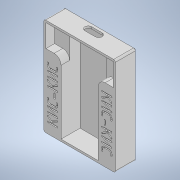
# Autodesk Inventor part: Корпус
Saved by Autodesk Inventor 2021.2 (Build 252289000, 289)
## iProperties
Created: 2023-10-18
Part Number: Корпус
Material: Типовые
Document SubType Name: Modeling
Designer: DELL
Density: 1 g/cm^3
Appearance: По умолчанию
Author: DELL
Autodesk Inventor part; units mm, degrees
ref_plane "YZ Plane" through (0, 0, 0) normal (1, 0, 0) x (0, 1, 0)
ref_plane "XZ Plane" through (0, 0, 0) normal (0, 1, 0) x (-1, 0, 0)
ref_plane "XY Plane" through (0, 0, 0) normal (0, 0, 1) x (1, 0, 0)
sketch "Эскиз1" plane through (0, 0, 0) normal (0, 0, 1) x (1, 0, 0)
  line L0 (10.25, -26.5) -> (-10.25, -26.5) construction
  line L1 (-10.25, -26.5) -> (-10.25, 26.5) construction
  line L2 (-10.25, 26.5) -> (10.25, 26.5) construction
  line L3 (10.25, 26.5) -> (10.25, -26.5) construction
  line L4 (10.25, -26.5) -> (-10.25, 26.5) construction
  line L5 (-10.25, -26.5) -> (10.25, 26.5) construction
  line L6 (19, 14.5) -> (-19, 14.5) construction
  line L7 (-19, 14.5) -> (-19, 26.5) construction
  line L8 (-19, 26.5) -> (19, 26.5) construction
  line L9 (19, 26.5) -> (19, 14.5) construction
  line L10 (19, 14.5) -> (-19, 26.5) construction
  line L11 (-19, 14.5) -> (19, 26.5) construction
  line L12 (-19.5, 14) -> (-14.75, 14)
  arc A0 (-10.75, 10) -> (-14.75, 14) centre (-14.75, 10) ccw
  line L13 (-10.75, 10) -> (-10.75, -27)
  line L14 (-10.75, -27) -> (10.75, -27)
  line L15 (10.75, -27) -> (10.75, 10)
  arc A1 (14.75, 14) -> (10.75, 10) centre (14.75, 10) ccw
  line L16 (14.75, 14) -> (19.5, 14)
  line L17 (19.5, 14) -> (19.5, 27)
  line L18 (19.5, 27) -> (-19.5, 27)
  line L19 (-19.5, 27) -> (-19.5, 14)
  line L20 (0, 26.5) -> (0, -26.5) construction
  line L21 (20.7, -28.2) -> (-20.7, -28.2)
  line L22 (-20.7, -28.2) -> (-20.7, 28.2)
  line L23 (-20.7, 28.2) -> (20.7, 28.2)
  line L24 (20.7, 28.2) -> (20.7, -28.2)
  line L25 (20.7, -28.2) -> (-20.7, 28.2) construction
  line L26 (-20.7, -28.2) -> (20.7, 28.2) construction
  line L27 (-10.75, 10) -> (-10.75, 27)
  line L28 (10.75, 10) -> (10.75, 27)
  point P0 (0, 0)
  point P1 (0, 20.5)
  point P2 (0, 20.5)
  point P3 (0, 0)
  point P4 (0, 0)
  dimension "d0" = 20.5
  dimension "d1" = 53
  dimension "d2" = 38
  dimension "d3" = 12
  dimension "d4" = 0
  dimension "d5" = 0.5
  dimension "d8" = 0.5
  dimension "d9" = 0.5
  dimension "d10" = 0.5
  dimension "d11" = 0.5
  dimension "d12" = 4
  dimension "d13" = 1.2
  dimension "d14" = 1.2
  dimension "d15" = 1.2
  constraints: 58 end point, 11 midpoint, 10 perpendicular, 7 parallel, 5 horizontal, 4 point on circle, 4 tangent, 3 point on line, 2 centre point, 1 vertical alignment, 3 other
  measures "d0" distance of L1.end L2.end
  measures "d1" distance of L0.end L1.end
  measures "d2" distance of L7.end L8.end
  measures "d3" distance of L6.end L7.end
  measures "d4" distance between parallel lines of L2 L8
  measures "d5" distance between parallel lines of L19 L7
  measures "d8" distance between parallel lines of L18 L8
  measures "d9" distance between parallel lines of L6 L12
  measures "d10" distance between parallel lines of L1 L13
  measures "d11" distance between parallel lines of L0 L14
  measures "d12" radius of A0
  measures "d13" distance between parallel lines of L23 L18
  measures "d14" distance between parallel lines of L22 L19
  measures "d15" distance between parallel lines of L14 L21
extrude "Выдавливание1" add sketch "Эскиз1" along normal blind 6 contours L19 L18 L27 A0 L12 | L18 L17 L16 A1 L28 | L21 L22 L23 L24
extrude "Выдавливание2" add sketch "Эскиз1" along normal blind 5 from surface at 6
extrude "Выдавливание3" add sketch "Эскиз1" against normal blind 1 contours L19 L18 L27 A0 L12 | L27 L18 L28 L15 L14 L13 | L18 L17 L16 A1 L28 | L21 L22 L23 L24
fillet "Сопряжение1" radius 1 4 edges at (-20.7, 28.2, 5) (20.7, 28.2, 5) (-20.7, -28.2, 5) (20.7, -28.2, 5)
chamfer "Фаска1" distance 0.5 angle 45 8 edges at (20.7, 0, -1) (20.4071, -27.9071, -1) (0, -28.2, -1) (-20.4071, -27.9071, -1) (-20.7, 0, -1) (-20.4071, 27.9071, -1) (0, 28.2, -1) (20.4071, 27.9071, -1)
sketch "Эскиз2" plane through (-19.7, 28.2, 11) normal (0, 1, 0) x (1, 0, 0)
  line L0 (8.95, 11) -> (30.45, 11) construction
  line L1 (8.95, 11) -> (8.95, 5) construction
  line L2 (30.45, 11) -> (30.45, 5) construction
  line L3 (22.7, 8) -> (16.7, 8) construction
  line L4 (22.7, 10) -> (16.7, 10)
  line L5 (16.7, 6) -> (22.7, 6)
  arc A0 (22.7, 6) -> (22.7, 10) centre (22.7, 8) ccw
  arc A1 (16.7, 10) -> (16.7, 6) centre (16.7, 8) ccw
  point P0 (19.7, 11)
  point P1 (19.7, 8)
  point P2 (19.7, 11)
  dimension "d26" = 10
  dimension "d27" = 4
  dimension "d28" = 1
  constraints: 8 end point, 4 point on circle, 4 tangent, 2 centre point, 2 midpoint, 2 parallel, 1 vertical alignment
  measures "d27" distance between parallel lines of L5 L4
  measures "d28" distance between parallel lines of L4 L0
extrude "Выдавливание4" cut sketch "Эскиз2" against normal up to next
sketch "Эскиз3" plane through (-19.7, 28.2, 11) normal (0, 0, 1) x (1, 0, 0)
  line L0 (38.4355, -18.4335) -> (38.4355, -51.3182) construction
  line L1 (38.4355, -51.3182) -> (33.2904, -51.3182) construction
  line L2 (33.2904, -51.3182) -> (33.2904, -18.4335) construction
  line L3 (33.2904, -18.4335) -> (38.4355, -18.4335) construction
  line L4 (0.9645, -51.3182) -> (0.9645, -18.4335) construction
  line L5 (0.9645, -18.4335) -> (6.1096, -18.4335) construction
  line L6 (6.1096, -18.4335) -> (6.1096, -51.3182) construction
  line L7 (6.1096, -51.3182) -> (0.9645, -51.3182) construction
  line L8 (39.4, -56.4) -> (0, -56.4) construction
  line L9 (19.7, -56.4) -> (19.7, 0) construction
  line L10 (16.7, 0) -> (22.7, 0) construction
  line L11 (35.4384, -20.4584) -> (34.6425, -19.7935)
  line L12 (34.6425, -19.7935) -> (32.7183, -19.7935)
  spline S0 degree 2 poles (32.7183, -19.7935) (32.3355, -19.7935) (32.3355, -19.4107) knots 0 0 0 1 1 1
  spline S1 degree 2 poles (32.3355, -19.4107) (32.3355, -19.0279) (32.7183, -19.0279) knots 0 0 0 1 1 1
  line L13 (32.7183, -19.0279) -> (38.0577, -19.0279)
  spline S2 degree 2 poles (38.0577, -19.0279) (38.4355, -19.0279) (38.4355, -19.4107) knots 0 0 0 1 1 1
  spline S3 degree 2 poles (38.4355, -19.4107) (38.4355, -19.7935) (38.0577, -19.7935) knots 0 0 0 1 1 1
  line L14 (38.0577, -19.7935) -> (35.65, -19.7935)
  line L15 (35.65, -19.7935) -> (38.3096, -22.0905)
  spline S4 degree 2 poles (38.3096, -22.0905) (38.4355, -22.2013) (38.4355, -22.3776) knots 0 0 0 1 1 1
  spline S5 degree 2 poles (38.4355, -22.3776) (38.4355, -22.7604) (38.0577, -22.7604) knots 0 0 0 1 1 1
  spline S6 degree 2 poles (38.0577, -22.7604) (37.9116, -22.7604) (37.7706, -22.5338) knots 0 0 0 1 1 1
  line L16 (37.7706, -22.5338) -> (35.9774, -20.9823)
  line L17 (35.9774, -20.9823) -> (32.9047, -22.705)
  spline S7 degree 2 poles (32.9047, -22.705) (32.814, -22.7604) (32.7183, -22.7604) knots 0 0 0 1 1 1
  spline S8 degree 2 poles (32.7183, -22.7604) (32.5672, -22.7604) (32.3355, -22.5237) (32.3355, -22.3776) knots 0 0 0 1 2 2 2
  spline S9 degree 2 poles (32.3355, -22.3776) (32.3355, -22.1459) (32.5823, -22.025) knots 0 0 0 1 1 1
  line L18 (32.5823, -22.025) -> (35.4384, -20.4584)
  spline S10 degree 2 poles (38.4355, -27.1226) (38.4355, -27.5054) (38.0577, -27.5054) knots 0 0 0 1 1 1
  line L19 (38.0577, -27.5054) -> (32.7183, -27.5054)
  spline S11 degree 2 poles (32.7183, -27.5054) (32.3355, -27.5054) (32.3355, -27.1226) knots 0 0 0 1 1 1
  spline S12 degree 2 poles (32.3355, -27.1226) (32.3355, -26.7398) (32.7183, -26.7398) knots 0 0 0 1 1 1
  line L20 (32.7183, -26.7398) -> (36.5869, -26.7398)
  line L21 (36.5869, -26.7398) -> (32.9903, -24.5436)
  spline S13 degree 2 poles (32.9903, -24.5436) (32.6881, -24.5436) (32.5874, -24.5134) knots 0 0 0 1 1 1
  spline S14 degree 2 poles (32.5874, -24.5134) (32.3355, -24.4479) (32.3355, -24.1608) knots 0 0 0 1 1 1
  spline S15 degree 2 poles (32.3355, -24.1608) (32.3355, -23.7779) (32.7183, -23.7779) knots 0 0 0 1 1 1
  line L22 (32.7183, -23.7779) -> (38.0577, -23.7779)
  spline S16 degree 2 poles (38.0577, -23.7779) (38.4355, -23.7779) (38.4355, -24.1608) knots 0 0 0 1 1 1
  spline S17 degree 2 poles (38.4355, -24.1608) (38.4355, -24.5436) (38.0577, -24.5436) knots 0 0 0 1 1 1
  line L23 (38.0577, -24.5436) -> (34.1892, -24.5436)
  line L24 (34.1892, -24.5436) -> (37.7857, -26.7398)
  spline S18 degree 2 poles (37.7857, -26.7398) (38.0879, -26.7398) (38.1836, -26.765) knots 0 0 0 1 1 1
  spline S19 degree 2 poles (38.1836, -26.765) (38.4355, -26.8305) (38.4355, -27.1226) knots 0 0 0 1 1 1
  spline S20 degree 2 poles (38.4355, -31.2833) (38.4355, -31.6661) (38.0577, -31.6661) knots 0 0 0 1 1 1
  spline S21 degree 2 poles (38.0577, -31.6661) (37.6749, -31.6661) (37.6749, -31.2833) knots 0 0 0 1 1 1
  line L25 (37.6749, -31.2833) -> (37.6749, -30.0996)
  spline S22 degree 2 poles (37.6749, -30.0996) (37.6749, -29.6362) (37.277, -29.4044) knots 0 0 0 1 1 1
  spline S23 degree 2 poles (37.277, -29.4044) (37.0906, -29.2936) (36.8689, -29.2936) knots 0 0 0 1 1 1
  line L26 (36.8689, -29.2936) -> (33.9071, -29.2936)
  spline S24 degree 2 poles (33.9071, -29.2936) (33.5696, -29.2936) (33.0961, -29.7671) (33.0961, -30.0996) knots 0 0 0 1 2 2 2
  line L27 (33.0961, -30.0996) -> (33.0961, -31.2833)
  spline S25 degree 2 poles (33.0961, -31.2833) (33.0961, -31.6661) (32.7183, -31.6661) knots 0 0 0 1 1 1
  spline S26 degree 2 poles (32.7183, -31.6661) (32.3355, -31.6661) (32.3355, -31.2833) knots 0 0 0 1 1 1
  line L28 (32.3355, -31.2833) -> (32.3355, -30.0996)
  spline S27 degree 2 poles (32.3355, -30.0996) (32.3355, -29.4447) (33.2523, -28.528) (33.9071, -28.528) knots 0 0 0 1 2 2 2
  line L29 (33.9071, -28.528) -> (36.874, -28.528)
  spline S28 degree 2 poles (36.874, -28.528) (37.5187, -28.528) (38.4355, -29.4447) (38.4355, -30.0996) knots 0 0 0 1 2 2 2
  line L30 (38.4355, -30.0996) -> (38.4355, -31.2833)
  line L31 (33.8164, -35.439) -> (33.8164, -33.0665)
  spline S29 degree 2 poles (33.8164, -33.0665) (33.8164, -32.6836) (34.1993, -32.6836) knots 0 0 0 1 1 1
  spline S30 degree 2 poles (34.1993, -32.6836) (34.577, -32.6836) (34.577, -33.0665) knots 0 0 0 1 1 1
  line L32 (34.577, -33.0665) -> (34.577, -35.439)
  spline S31 degree 2 poles (34.577, -35.439) (34.577, -35.8218) (34.1993, -35.8218) knots 0 0 0 1 1 1
  spline S32 degree 2 poles (34.1993, -35.8218) (33.8164, -35.8218) (33.8164, -35.439) knots 0 0 0 1 1 1
  line L33 (35.4384, -38.2698) -> (34.6425, -37.6049)
  line L34 (34.6425, -37.6049) -> (32.7183, -37.6049)
  spline S33 degree 2 poles (32.7183, -37.6049) (32.3355, -37.6049) (32.3355, -37.2221) knots 0 0 0 1 1 1
  spline S34 degree 2 poles (32.3355, -37.2221) (32.3355, -36.8393) (32.7183, -36.8393) knots 0 0 0 1 1 1
  line L35 (32.7183, -36.8393) -> (38.0577, -36.8393)
  spline S35 degree 2 poles (38.0577, -36.8393) (38.4355, -36.8393) (38.4355, -37.2221) knots 0 0 0 1 1 1
  spline S36 degree 2 poles (38.4355, -37.2221) (38.4355, -37.6049) (38.0577, -37.6049) knots 0 0 0 1 1 1
  line L36 (38.0577, -37.6049) -> (35.65, -37.6049)
  line L37 (35.65, -37.6049) -> (38.3096, -39.9019)
  spline S37 degree 2 poles (38.3096, -39.9019) (38.4355, -40.0127) (38.4355, -40.189) knots 0 0 0 1 1 1
  spline S38 degree 2 poles (38.4355, -40.189) (38.4355, -40.5718) (38.0577, -40.5718) knots 0 0 0 1 1 1
  spline S39 degree 2 poles (38.0577, -40.5718) (37.9116, -40.5718) (37.7706, -40.3452) knots 0 0 0 1 1 1
  line L38 (37.7706, -40.3452) -> (35.9774, -38.7937)
  line L39 (35.9774, -38.7937) -> (32.9047, -40.5164)
  spline S40 degree 2 poles (32.9047, -40.5164) (32.814, -40.5718) (32.7183, -40.5718) knots 0 0 0 1 1 1
  spline S41 degree 2 poles (32.7183, -40.5718) (32.5672, -40.5718) (32.3355, -40.3351) (32.3355, -40.189) knots 0 0 0 1 2 2 2
  spline S42 degree 2 poles (32.3355, -40.189) (32.3355, -39.9573) (32.5823, -39.8364) knots 0 0 0 1 1 1
  line L40 (32.5823, -39.8364) -> (35.4384, -38.2698)
  spline S43 degree 2 poles (38.4355, -44.934) (38.4355, -45.3168) (38.0577, -45.3168) knots 0 0 0 1 1 1
  line L41 (38.0577, -45.3168) -> (32.7183, -45.3168)
  spline S44 degree 2 poles (32.7183, -45.3168) (32.3355, -45.3168) (32.3355, -44.934) knots 0 0 0 1 1 1
  spline S45 degree 2 poles (32.3355, -44.934) (32.3355, -44.5512) (32.7183, -44.5512) knots 0 0 0 1 1 1
  line L42 (32.7183, -44.5512) -> (36.5869, -44.5512)
  line L43 (36.5869, -44.5512) -> (32.9903, -42.355)
  spline S46 degree 2 poles (32.9903, -42.355) (32.6881, -42.355) (32.5874, -42.3248) knots 0 0 0 1 1 1
  spline S47 degree 2 poles (32.5874, -42.3248) (32.3355, -42.2593) (32.3355, -41.9722) knots 0 0 0 1 1 1
  spline S48 degree 2 poles (32.3355, -41.9722) (32.3355, -41.5893) (32.7183, -41.5893) knots 0 0 0 1 1 1
  line L44 (32.7183, -41.5893) -> (38.0577, -41.5893)
  spline S49 degree 2 poles (38.0577, -41.5893) (38.4355, -41.5893) (38.4355, -41.9722) knots 0 0 0 1 1 1
  spline S50 degree 2 poles (38.4355, -41.9722) (38.4355, -42.355) (38.0577, -42.355) knots 0 0 0 1 1 1
  line L45 (38.0577, -42.355) -> (34.1892, -42.355)
  line L46 (34.1892, -42.355) -> (37.7857, -44.5512)
  spline S51 degree 2 poles (37.7857, -44.5512) (38.0879, -44.5512) (38.1836, -44.5764) knots 0 0 0 1 1 1
  spline S52 degree 2 poles (38.1836, -44.5764) (38.4355, -44.6419) (38.4355, -44.934) knots 0 0 0 1 1 1
  spline S53 degree 2 poles (38.4355, -49.0947) (38.4355, -49.4775) (38.0577, -49.4775) knots 0 0 0 1 1 1
  spline S54 degree 2 poles (38.0577, -49.4775) (37.6749, -49.4775) (37.6749, -49.0947) knots 0 0 0 1 1 1
  line L47 (37.6749, -49.0947) -> (37.6749, -47.911)
  spline S55 degree 2 poles (37.6749, -47.911) (37.6749, -47.4475) (37.277, -47.2158) knots 0 0 0 1 1 1
  spline S56 degree 2 poles (37.277, -47.2158) (37.0906, -47.105) (36.8689, -47.105) knots 0 0 0 1 1 1
  line L48 (36.8689, -47.105) -> (33.9071, -47.105)
  spline S57 degree 2 poles (33.9071, -47.105) (33.5696, -47.105) (33.0961, -47.5785) (33.0961, -47.911) knots 0 0 0 1 2 2 2
  line L49 (33.0961, -47.911) -> (33.0961, -49.0947)
  spline S58 degree 2 poles (33.0961, -49.0947) (33.0961, -49.4775) (32.7183, -49.4775) knots 0 0 0 1 1 1
  spline S59 degree 2 poles (32.7183, -49.4775) (32.3355, -49.4775) (32.3355, -49.0947) knots 0 0 0 1 1 1
  line L50 (32.3355, -49.0947) -> (32.3355, -47.911)
  spline S60 degree 2 poles (32.3355, -47.911) (32.3355, -47.2561) (33.2523, -46.3394) (33.9071, -46.3394) knots 0 0 0 1 2 2 2
  line L51 (33.9071, -46.3394) -> (36.874, -46.3394)
  spline S61 degree 2 poles (36.874, -46.3394) (37.5187, -46.3394) (38.4355, -47.2561) (38.4355, -47.911) knots 0 0 0 1 2 2 2
  line L52 (38.4355, -47.911) -> (38.4355, -49.0947)
  line L53 (3.9616, -49.2932) -> (4.7575, -49.9582)
  line L54 (4.7575, -49.9582) -> (6.6817, -49.9582)
  spline S62 degree 2 poles (6.6817, -49.9582) (7.0645, -49.9582) (7.0645, -50.341) knots 0 0 0 1 1 1
  spline S63 degree 2 poles (7.0645, -50.341) (7.0645, -50.7238) (6.6817, -50.7238) knots 0 0 0 1 1 1
  line L55 (6.6817, -50.7238) -> (1.3423, -50.7238)
  spline S64 degree 2 poles (1.3423, -50.7238) (0.9645, -50.7238) (0.9645, -50.341) knots 0 0 0 1 1 1
  spline S65 degree 2 poles (0.9645, -50.341) (0.9645, -49.9582) (1.3423, -49.9582) knots 0 0 0 1 1 1
  line L56 (1.3423, -49.9582) -> (3.75, -49.9582)
  line L57 (3.75, -49.9582) -> (1.0904, -47.6612)
  spline S66 degree 2 poles (1.0904, -47.6612) (0.9645, -47.5504) (0.9645, -47.3741) knots 0 0 0 1 1 1
  spline S67 degree 2 poles (0.9645, -47.3741) (0.9645, -46.9913) (1.3423, -46.9913) knots 0 0 0 1 1 1
  spline S68 degree 2 poles (1.3423, -46.9913) (1.4884, -46.9913) (1.6294, -47.2179) knots 0 0 0 1 1 1
  line L58 (1.6294, -47.2179) -> (3.4226, -48.7694)
  line L59 (3.4226, -48.7694) -> (6.4953, -47.0467)
  spline S69 degree 2 poles (6.4953, -47.0467) (6.586, -46.9913) (6.6817, -46.9913) knots 0 0 0 1 1 1
  spline S70 degree 2 poles (6.6817, -46.9913) (6.8328, -46.9913) (7.0645, -47.228) (7.0645, -47.3741) knots 0 0 0 1 2 2 2
  spline S71 degree 2 poles (7.0645, -47.3741) (7.0645, -47.6058) (6.8177, -47.7267) knots 0 0 0 1 1 1
  line L60 (6.8177, -47.7267) -> (3.9616, -49.2932)
  spline S72 degree 2 poles (0.9645, -42.6291) (0.9645, -42.2463) (1.3423, -42.2463) knots 0 0 0 1 1 1
  line L61 (1.3423, -42.2463) -> (6.6817, -42.2463)
  spline S73 degree 2 poles (6.6817, -42.2463) (7.0645, -42.2463) (7.0645, -42.6291) knots 0 0 0 1 1 1
  spline S74 degree 2 poles (7.0645, -42.6291) (7.0645, -43.0119) (6.6817, -43.0119) knots 0 0 0 1 1 1
  line L62 (6.6817, -43.0119) -> (2.8131, -43.0119)
  line L63 (2.8131, -43.0119) -> (6.4097, -45.2081)
  spline S75 degree 2 poles (6.4097, -45.2081) (6.7119, -45.2081) (6.8126, -45.2383) knots 0 0 0 1 1 1
  spline S76 degree 2 poles (6.8126, -45.2383) (7.0645, -45.3038) (7.0645, -45.5909) knots 0 0 0 1 1 1
  spline S77 degree 2 poles (7.0645, -45.5909) (7.0645, -45.9738) (6.6817, -45.9738) knots 0 0 0 1 1 1
  line L64 (6.6817, -45.9738) -> (1.3423, -45.9738)
  spline S78 degree 2 poles (1.3423, -45.9738) (0.9645, -45.9738) (0.9645, -45.5909) knots 0 0 0 1 1 1
  spline S79 degree 2 poles (0.9645, -45.5909) (0.9645, -45.2081) (1.3423, -45.2081) knots 0 0 0 1 1 1
  line L65 (1.3423, -45.2081) -> (5.2108, -45.2081)
  line L66 (5.2108, -45.2081) -> (1.6143, -43.0119)
  spline S80 degree 2 poles (1.6143, -43.0119) (1.3121, -43.0119) (1.2164, -42.9867) knots 0 0 0 1 1 1
  spline S81 degree 2 poles (1.2164, -42.9867) (0.9645, -42.9212) (0.9645, -42.6291) knots 0 0 0 1 1 1
  spline S82 degree 2 poles (0.9645, -38.4684) (0.9645, -38.0856) (1.3423, -38.0856) knots 0 0 0 1 1 1
  spline S83 degree 2 poles (1.3423, -38.0856) (1.7251, -38.0856) (1.7251, -38.4684) knots 0 0 0 1 1 1
  line L67 (1.7251, -38.4684) -> (1.7251, -39.6521)
  spline S84 degree 2 poles (1.7251, -39.6521) (1.7251, -40.1155) (2.123, -40.3473) knots 0 0 0 1 1 1
  spline S85 degree 2 poles (2.123, -40.3473) (2.3094, -40.4581) (2.5311, -40.4581) knots 0 0 0 1 1 1
  line L68 (2.5311, -40.4581) -> (5.4929, -40.4581)
  spline S86 degree 2 poles (5.4929, -40.4581) (5.8304, -40.4581) (6.3039, -39.9846) (6.3039, -39.6521) knots 0 0 0 1 2 2 2
  line L69 (6.3039, -39.6521) -> (6.3039, -38.4684)
  spline S87 degree 2 poles (6.3039, -38.4684) (6.3039, -38.0856) (6.6817, -38.0856) knots 0 0 0 1 1 1
  spline S88 degree 2 poles (6.6817, -38.0856) (7.0645, -38.0856) (7.0645, -38.4684) knots 0 0 0 1 1 1
  line L70 (7.0645, -38.4684) -> (7.0645, -39.6521)
  spline S89 degree 2 poles (7.0645, -39.6521) (7.0645, -40.307) (6.1477, -41.2237) (5.4929, -41.2237) knots 0 0 0 1 2 2 2
  line L71 (5.4929, -41.2237) -> (2.526, -41.2237)
  spline S90 degree 2 poles (2.526, -41.2237) (1.8813, -41.2237) (0.9645, -40.307) (0.9645, -39.6521) knots 0 0 0 1 2 2 2
  line L72 (0.9645, -39.6521) -> (0.9645, -38.4684)
  line L73 (5.5836, -34.3127) -> (5.5836, -36.6852)
  spline S91 degree 2 poles (5.5836, -36.6852) (5.5836, -37.0681) (5.2007, -37.0681) knots 0 0 0 1 1 1
  spline S92 degree 2 poles (5.2007, -37.0681) (4.823, -37.0681) (4.823, -36.6852) knots 0 0 0 1 1 1
  line L74 (4.823, -36.6852) -> (4.823, -34.3127)
  spline S93 degree 2 poles (4.823, -34.3127) (4.823, -33.9299) (5.2007, -33.9299) knots 0 0 0 1 1 1
  spline S94 degree 2 poles (5.2007, -33.9299) (5.5836, -33.9299) (5.5836, -34.3127) knots 0 0 0 1 1 1
  line L75 (3.9616, -31.4819) -> (4.7575, -32.1468)
  line L76 (4.7575, -32.1468) -> (6.6817, -32.1468)
  spline S95 degree 2 poles (6.6817, -32.1468) (7.0645, -32.1468) (7.0645, -32.5296) knots 0 0 0 1 1 1
  spline S96 degree 2 poles (7.0645, -32.5296) (7.0645, -32.9124) (6.6817, -32.9124) knots 0 0 0 1 1 1
  line L77 (6.6817, -32.9124) -> (1.3423, -32.9124)
  spline S97 degree 2 poles (1.3423, -32.9124) (0.9645, -32.9124) (0.9645, -32.5296) knots 0 0 0 1 1 1
  spline S98 degree 2 poles (0.9645, -32.5296) (0.9645, -32.1468) (1.3423, -32.1468) knots 0 0 0 1 1 1
  line L78 (1.3423, -32.1468) -> (3.75, -32.1468)
  line L79 (3.75, -32.1468) -> (1.0904, -29.8498)
  spline S99 degree 2 poles (1.0904, -29.8498) (0.9645, -29.739) (0.9645, -29.5627) knots 0 0 0 1 1 1
  spline S100 degree 2 poles (0.9645, -29.5627) (0.9645, -29.1799) (1.3423, -29.1799) knots 0 0 0 1 1 1
  spline S101 degree 2 poles (1.3423, -29.1799) (1.4884, -29.1799) (1.6294, -29.4065) knots 0 0 0 1 1 1
  line L80 (1.6294, -29.4065) -> (3.4226, -30.958)
  line L81 (3.4226, -30.958) -> (6.4953, -29.2353)
  spline S102 degree 2 poles (6.4953, -29.2353) (6.586, -29.1799) (6.6817, -29.1799) knots 0 0 0 1 1 1
  spline S103 degree 2 poles (6.6817, -29.1799) (6.8328, -29.1799) (7.0645, -29.4166) (7.0645, -29.5627) knots 0 0 0 1 2 2 2
  spline S104 degree 2 poles (7.0645, -29.5627) (7.0645, -29.7944) (6.8177, -29.9153) knots 0 0 0 1 1 1
  line L82 (6.8177, -29.9153) -> (3.9616, -31.4819)
  spline S105 degree 2 poles (0.9645, -24.8177) (0.9645, -24.4349) (1.3423, -24.4349) knots 0 0 0 1 1 1
  line L83 (1.3423, -24.4349) -> (6.6817, -24.4349)
  spline S106 degree 2 poles (6.6817, -24.4349) (7.0645, -24.4349) (7.0645, -24.8177) knots 0 0 0 1 1 1
  spline S107 degree 2 poles (7.0645, -24.8177) (7.0645, -25.2005) (6.6817, -25.2005) knots 0 0 0 1 1 1
  line L84 (6.6817, -25.2005) -> (2.8131, -25.2005)
  line L85 (2.8131, -25.2005) -> (6.4097, -27.3967)
  spline S108 degree 2 poles (6.4097, -27.3967) (6.7119, -27.3967) (6.8126, -27.4269) knots 0 0 0 1 1 1
  spline S109 degree 2 poles (6.8126, -27.4269) (7.0645, -27.4924) (7.0645, -27.7795) knots 0 0 0 1 1 1
  spline S110 degree 2 poles (7.0645, -27.7795) (7.0645, -28.1624) (6.6817, -28.1624) knots 0 0 0 1 1 1
  line L86 (6.6817, -28.1624) -> (1.3423, -28.1624)
  spline S111 degree 2 poles (1.3423, -28.1624) (0.9645, -28.1624) (0.9645, -27.7795) knots 0 0 0 1 1 1
  spline S112 degree 2 poles (0.9645, -27.7795) (0.9645, -27.3967) (1.3423, -27.3967) knots 0 0 0 1 1 1
  line L87 (1.3423, -27.3967) -> (5.2108, -27.3967)
  line L88 (5.2108, -27.3967) -> (1.6143, -25.2005)
  spline S113 degree 2 poles (1.6143, -25.2005) (1.3121, -25.2005) (1.2164, -25.1753) knots 0 0 0 1 1 1
  spline S114 degree 2 poles (1.2164, -25.1753) (0.9645, -25.1098) (0.9645, -24.8177) knots 0 0 0 1 1 1
  spline S115 degree 2 poles (0.9645, -20.657) (0.9645, -20.2742) (1.3423, -20.2742) knots 0 0 0 1 1 1
  spline S116 degree 2 poles (1.3423, -20.2742) (1.7251, -20.2742) (1.7251, -20.657) knots 0 0 0 1 1 1
  line L89 (1.7251, -20.657) -> (1.7251, -21.8407)
  spline S117 degree 2 poles (1.7251, -21.8407) (1.7251, -22.3041) (2.123, -22.5359) knots 0 0 0 1 1 1
  spline S118 degree 2 poles (2.123, -22.5359) (2.3094, -22.6467) (2.5311, -22.6467) knots 0 0 0 1 1 1
  line L90 (2.5311, -22.6467) -> (5.4929, -22.6467)
  spline S119 degree 2 poles (5.4929, -22.6467) (5.8304, -22.6467) (6.3039, -22.1732) (6.3039, -21.8407) knots 0 0 0 1 2 2 2
  line L91 (6.3039, -21.8407) -> (6.3039, -20.657)
  spline S120 degree 2 poles (6.3039, -20.657) (6.3039, -20.2742) (6.6817, -20.2742) knots 0 0 0 1 1 1
  spline S121 degree 2 poles (6.6817, -20.2742) (7.0645, -20.2742) (7.0645, -20.657) knots 0 0 0 1 1 1
  line L92 (7.0645, -20.657) -> (7.0645, -21.8407)
  spline S122 degree 2 poles (7.0645, -21.8407) (7.0645, -22.4956) (6.1477, -23.4123) (5.4929, -23.4123) knots 0 0 0 1 2 2 2
  line L93 (5.4929, -23.4123) -> (2.526, -23.4123)
  spline S123 degree 2 poles (2.526, -23.4123) (1.8813, -23.4123) (0.9645, -22.4956) (0.9645, -21.8407) knots 0 0 0 1 2 2 2
  line L94 (0.9645, -21.8407) -> (0.9645, -20.657)
  point P0 (19.7, -28.2)
  constraints: 2 end point, 2 midpoint, 8 other
emboss "Рельеф1" sketch "Эскиз3" operation cut depth 0.6 direction (0, 0, -1)
equation "\"d8\" = d5"
equation "\"d9\" = d5"
equation "\"d10\" = d5"
equation "\"d11\" = d5"
equation "\"d14\" = d13"
equation "\"d15\" = d13"
